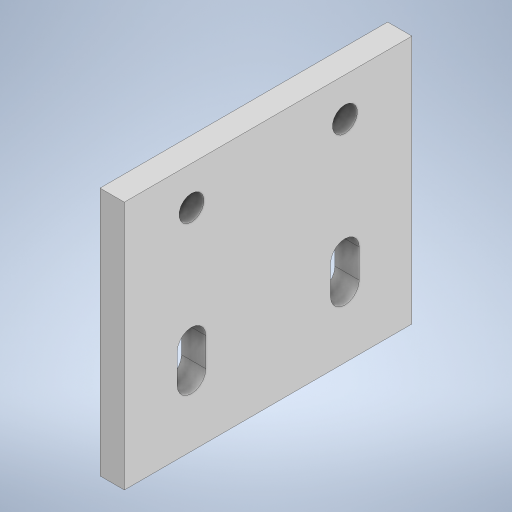
# Autodesk Inventor part: mounting bracket 1
Saved by Autodesk Inventor 2023 (Build 270158000, 158)
## iProperties
Created: 2023-02-02
Part Number: mounting bracket 1
Material: Generic
Document SubType Name: Modeling
Designer: Steven
Density: 1 g/cm^3
Appearance: Default
Author: Steven
Autodesk Inventor part; units mm, degrees
ref_plane "YZ Plane" through (0, 0, 0) normal (1, 0, 0) x (0, 1, 0)
ref_plane "XZ Plane" through (0, 0, 0) normal (0, 1, 0) x (-1, 0, 0)
ref_plane "XY Plane" through (0, 0, 0) normal (0, 0, 1) x (1, 0, 0)
sketch "Sketch1" plane through (0, 0, 0) normal (1, 0, 0) x (0, 1, 0)
  line L0 (0, 0) -> (-65, 0)
  line L1 (-65, 0) -> (-65, -75)
  line L2 (-65, -75) -> (0, -75)
  line L3 (0, -75) -> (0, 0)
  line L4 (-40.75, -13.75) -> (-48.25, -13.75)
  line L5 (-48.25, -13.75) -> (-48.25, -21.25)
  line L6 (-48.25, -21.25) -> (-40.75, -21.25)
  line L7 (-40.75, -21.25) -> (-40.75, -13.75)
  arc A0 (-40.75, -21.25) -> (-40.75, -13.75) centre (-40.75, -17.5) ccw
  arc A1 (-48.25, -13.75) -> (-48.25, -21.25) centre (-48.25, -17.5) ccw
  line L8 (-40.75, -53.75) -> (-48.25, -53.75)
  line L9 (-48.25, -53.75) -> (-48.25, -61.25)
  line L10 (-48.25, -61.25) -> (-40.75, -61.25)
  line L11 (-40.75, -61.25) -> (-40.75, -53.75)
  arc A2 (-40.75, -61.25) -> (-40.75, -53.75) centre (-40.75, -57.5) ccw
  arc A3 (-48.25, -53.75) -> (-48.25, -61.25) centre (-48.25, -57.5) ccw
  circle A4 centre (-10, -17.5) radius 3.25
  circle A5 centre (-10, -57.5) radius 3.25
  dimension "d1" = 75
  dimension "d4" = 7.5
  dimension "d5" = 7.5
  dimension "d8" = 13.75
  dimension "d10" = 40
  dimension "d15" = 10
  dimension "d16" = 6.5
  dimension "d17" = 6.5
  dimension "d18" = 30.75
  dimension "d19" = 65
  dimension "d20" = 7.5
  constraints: 24 end point, 8 point on circle, 8 tangent, 6 centre point, 6 parallel, 4 midpoint, 3 horizontal, 3 perpendicular, 3 vertical alignment, 2 coincident, 2 horizontal alignment
  measures "d1" distance of L0.end L1.end
  measures "d4" distance between parallel lines of L6 L4
  measures "d5" distance between parallel lines of L10 L8
  measures "d8" distance between parallel lines of L0 L4
  measures "d10" distance of point (-40.75, -57.5) point (-40.75, -17.5)
  measures "d15" distance from line of L3 point (-10, -17.5)
  measures "d16" diameter of A4
  measures "d17" diameter of A5
  measures "d18" distance of A4.centre A0.centre
  measures "d19" distance between parallel lines of L1 L3
  measures "d20" distance of A1.centre A0.centre
extrude "Extrusion1" add sketch "Sketch1" along normal blind 6.35
equation "\"d5\" = d4"
equation "\"d8\" = -0.5 * d4 + 0.5 * d1 - 0.5 * d10"
equation "\"d17\" = d16"
body "Solid1"
